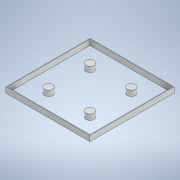
# Autodesk Inventor part: map1
Saved by Autodesk Inventor 2020 (Build 240168000, 168)
## iProperties
Created: 2020-04-02
Part Number: map1
Material: Generic
Document SubType Name: Modeling
Designer: Tarsoly
Density: 1 g/cm^3
Appearance: Default
Author: Tarsoly
Autodesk Inventor part; units mm, degrees
ref_plane "YZ Plane" through (0, 0, 0) normal (1, 0, 0) x (0, 1, 0)
ref_plane "XZ Plane" through (0, 0, 0) normal (0, 1, 0) x (-1, 0, 0)
ref_plane "XY Plane" through (0, 0, 0) normal (0, 0, 1) x (1, 0, 0)
sketch "Sketch1" plane through (0, 0, 0) normal (0, 1, 0) x (-1, 0, 0)
  line L0 (3000, -3000) -> (-3000, -3000)
  line L1 (-3000, -3000) -> (-3000, 3000)
  line L2 (-3000, 3000) -> (3000, 3000)
  line L3 (3000, 3000) -> (3000, -3000)
  line L4 (3000, -3000) -> (-3000, 3000) construction
  line L5 (-3000, -3000) -> (3000, 3000) construction
  line L6 (-3050, -3050) -> (3050, -3050)
  line L7 (3050, -3050) -> (3050, 3050)
  line L8 (3050, 3050) -> (-3050, 3050)
  line L9 (-3050, 3050) -> (-3050, -3050)
  circle A0 centre (1500, -1500) radius 300
  circle A1 centre (-1500, -1500) radius 300
  circle A2 centre (-1500, 1500) radius 300
  circle A3 centre (1500, 1500) radius 300
  line L10 (1500, -1500) -> (-1500, -1500) construction
  line L11 (-1500, 1500) -> (-1500, -1500) construction
  line L12 (-1500, 1500) -> (1500, 1500) construction
  line L13 (1500, 1500) -> (1500, -1500) construction
  point P0 (0, 0)
  dimension "d0" = 6000
  dimension "d1" = 6000
  dimension "d2" = 50
  dimension "d3" = 600
  dimension "d4" = 600
  dimension "d5" = 600
  dimension "d6" = 600
  dimension "d7" = 3000
  constraints: 28 end point, 4 centre point, 4 parallel, 4 perpendicular, 4 point on line, 2 horizontal, 2 midpoint, 3 other
  measures "d0" distance of L1.end L2.end
  measures "d1" distance of L0.end L1.end
  measures "d2" distance between parallel lines of L0 L6
  measures "d3" diameter of A0
  measures "d4" diameter of A1
  measures "d5" diameter of A2
  measures "d6" diameter of A3
  measures "d7" distance of L11.start L10.end
extrude "Extrusion1" add sketch "Sketch1" along normal blind 400
equation "\"d7\" = 0.5 * d1"
body "Solid1"
